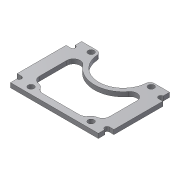
# Autodesk Inventor part: 付け根_サブフレーム_1_1
Saved by Autodesk Inventor 2017.3 (Build 213256000, 256)
## iProperties
Created: 2016-04-30
Part Number: 付け根_サブフレーム_1_1
Material: アルミニウム 2014-T4
Document SubType Name: Modeling
Designer: hiroaki
Density: 2.8 g/cm^3
Appearance: サテン
Mass: 3.21361 g
Surface Area: 17.5457 cm^2
Volume: 1.14772 cm^3
Author: hiroaki
Autodesk Inventor part; units mm, degrees
ref_plane "YZ Plane" through (0, 0, 0) normal (1, 0, 0) x (0, 1, 0)
ref_plane "XZ Plane" through (0, 0, 0) normal (0, 1, 0) x (-1, 0, 0)
ref_plane "XY Plane" through (0, 0, 0) normal (0, 0, 1) x (1, 0, 0)
sketch "スケッチ1" plane through (0, 0, 0) normal (0, 0, 1) x (1, 0, 0)
  circle A0 centre (0, 0) radius 10.5 construction
  line L0 (-13.5, -1) -> (13.5, -1) construction
  line L1 (13.5, -1) -> (13.5, -28) construction
  line L2 (13.5, -28) -> (-13.5, -28) construction
  line L3 (-13.5, -28) -> (-13.5, -1) construction
  circle A1 centre (-13.5, -1) radius 1.35
  circle A2 centre (13.5, -1) radius 1.35
  circle A3 centre (-13.5, -28) radius 1.35
  circle A4 centre (13.5, -28) radius 1.35
  line L4 (-19.75, 1) -> (-19.75, -1.9)
  line L5 (-19.75, -4) -> (-21.75, -4)
  line L6 (-21.75, -4) -> (-21.75, -26)
  line L7 (-21.75, -26) -> (-19.75, -26)
  line L8 (-19.75, -28.1) -> (-19.75, -31)
  line L9 (-19.75, -31) -> (19.75, -31)
  line L10 (19.75, -31) -> (19.75, -28.1)
  line L11 (19.75, -4) -> (21.75, -4)
  line L12 (21.75, -4) -> (21.75, -26)
  line L13 (21.75, -26) -> (19.75, -26)
  line L14 (0, 0) -> (0, -28) construction
  line L15 (-21.75, -15) -> (21.75, -15) construction
  arc A5 (-19.75, -4) -> (-19.75, -1.9) centre (-19.75, -2.95) ccw
  line L16 (-19.75, 1) -> (-10.9545, 1)
  circle A6 centre (-13.5, -1) radius 2 construction
  arc A7 (-19.75, -28.1) -> (-19.75, -26) centre (-19.75, -27.05) ccw
  arc A8 (19.75, -26) -> (19.75, -28.1) centre (19.75, -27.05) ccw
  line L17 (10.9545, 1) -> (19.75, 1)
  line L18 (19.75, 1) -> (19.75, -1.9)
  arc A9 (19.75, -1.9) -> (19.75, -4) centre (19.75, -2.95) ccw
  arc A10 (-10.9545, 1) -> (10.9545, 1) centre (0, 0) ccw
  point P0 (0, -1)
  dimension "d0" = 21
  dimension "d1" = 1
  dimension "d2" = 27
  dimension "d3" = 2.7
  dimension "d6" = 27
  dimension "d9" = 27
  dimension "d12" = 15
  dimension "d27" = 22
  dimension "d35" = 2
  dimension "d37" = 1.05
  dimension "d41" = 5
  dimension "d42" = 4
  dimension "d43" = 0.5
  dimension "d44" = 39.5
  constraints: 38 end point, 11 centre point, 10 perpendicular, 10 point on circle, 7 vertical alignment, 6 horizontal, 4 coincident, 4 midpoint, 4 symmetric about line, 3 vertical, 2 equal radius, 2 parallel, 2 tangent, 1 horizontal alignment, 7 other
  measures "d0" diameter of A0
  measures "d1" distance from line of point (0, 0) L0
  measures "d2" distance of L0.end L1.end
  measures "d3" diameter of A1
  measures "d6" distance of A1.centre A2.centre
  measures "d9" distance of A1.centre A3.centre
  measures "d12" distance from line of point (0, 0) L15
  measures "d27" distance of L5.end L6.end
  measures "d35" distance between parallel lines of L6 L4
  measures "d37" radius of A5
  measures "d41" distance from line of L4.start L5
  measures "d42" diameter of A6
  measures "d43" radial gap between concentric circles of A0 A10
  measures "d44" distance of L8.end L9.end
extrude "押し出し1" add sketch "スケッチ1" along normal blind 2
sketch "スケッチ2" plane through (0, 0, 2) normal (0, 0, 1) x (1, 0, 0)
  circle A0 centre (13.5, -28) radius 1.35 projected
  circle A1 centre (-13.5, -28) radius 1.35 projected
  circle A2 centre (13.5, -1) radius 1.35 projected
  circle A3 centre (-13.5, -1) radius 1.35 projected
  line L0 (-19.75, 1) -> (-19.75, -1.9) projected
  line L1 (-19.75, -31) -> (19.75, -31) projected
  arc A4 (-10.9545, 1) -> (10.9545, 1) centre (0, 0) ccw projected
  line L2 (-15.75, -2.9843) -> (-15.75, -25)
  line L3 (-15.75, -25) -> (-13.5, -25)
  arc A5 (-10.5, -28) -> (-13.5, -25) centre (-13.5, -28) ccw
  arc A6 (-15.75, -2.9843) -> (-12.4312, -3.8032) centre (-13.5, -1) ccw
  arc A7 (-12.4312, -3.8032) -> (12.4312, -3.8032) centre (0, 0) ccw
  arc A8 (12.4312, -3.8032) -> (15.75, -2.9843) centre (13.5, -1) ccw
  line L4 (15.75, -2.9843) -> (15.75, -25)
  line L5 (15.75, -25) -> (13.5, -25)
  arc A9 (13.5, -25) -> (10.5, -28) centre (13.5, -28) ccw
  line L6 (-10.5, -28) -> (10.5, -28)
  line L7 (0, 0) -> (0, -31) construction
  dimension "d47" = 3
  dimension "d48" = 4
  dimension "d49" = 2
  dimension "d50" = 3
  constraints: 12 end point, 10 point on circle, 5 centre point, 5 coincident, 3 equal radius, 2 perpendicular, 2 symmetric about line, 2 vertical, 1 midpoint, 1 parallel, 1 tangent
  measures "d47" radius of A5
  measures "d48" distance between parallel lines of L0 L2
  measures "d49" radial gap between concentric circles of A4 A7
  measures "d50" distance between parallel lines of L1 L6
extrude "押し出し2" cut sketch "スケッチ2" against normal blind 10 contours A6 A7 A8 L4 L5 A9 L6 A5 L3 L2
fillet "フィレット1" radius 3 8 edges at (-15.75, -2.9843, 1) (-12.4312, -3.8032, 1) (15.75, -2.9843, 1) (12.4312, -3.8032, 1) (-15.75, -25, 1) (-10.5, -28, 1) (15.75, -25, 1) (10.5, -28, 1)
fillet "フィレット1" radius 2 2 edges at (-10.9545, 1, 1) (10.9545, 1, 1)
equation "\"d6\" = d2"
equation "\"d9\" = d2"
equation "\"d12\" = d20"
equation "\"d27\" = d17"
equation "\"d41\" = d18"
equation "\"d17\" = 22"
equation "\"d18\" = 5"
equation "\"d20\" = 15"
